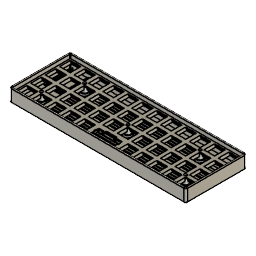
Like Planck (Autodesk Fusion 360 design; units mm, degrees)
Autodesk Fusion 360 part; units mm, degrees
note: some values were not read from the file. Set by a fixed rule: which sketch regions a step uses.
(part 1 of 2)
sketch "Base Sketch" plane through (0, 0, 0) normal (0, 0, 1) x (1, 0, 0)
  line L0 (99.1182, 9.2838) -> (99.1182, 3.0138)
  line L1 (104.144, 3.0138) -> (105.869, 3.0138)
  line L2 (105.869, 15.3128) -> (99.1182, 15.3128)
  line L3 (107.395, 2.7836) -> (121.394, 2.7836)
  line L4 (129.669, 12.0826) -> (129.669, 15.3128)
  line L5 (98.2941, 9.2838) -> (99.1182, 9.2838)
  line L6 (107.395, 16.7831) -> (107.395, 12.0826)
  line L7 (129.669, 9.2838) -> (130.495, 9.2838)
  line L8 (99.1182, 3.0138) -> (100.845, 3.0138)
  line L9 (130.495, 9.2838) -> (130.495, 12.0826)
  line L10 (0.0951, 0.2577) -> (0.0951, 76.4575)
  line L11 (122.92, 12.0826) -> (121.394, 12.0826)
  line L12 (2.6197, 16.7831) -> (16.6192, 16.7831)
  line L13 (121.394, 16.7831) -> (107.395, 16.7831)
  line L14 (105.869, 7.4827) -> (107.395, 7.4827)
  line L15 (228.695, 76.4575) -> (228.695, 0.2577)
  line L16 (105.869, 12.0826) -> (105.869, 15.3128)
  line L17 (98.2941, 12.0826) -> (98.2941, 9.2838)
  line L18 (107.395, 12.0826) -> (105.869, 12.0826)
  line L19 (121.394, 2.7836) -> (121.394, 7.4827)
  line L20 (124.645, 3.0138) -> (124.645, 1.8135)
  line L21 (99.1182, 12.0826) -> (98.2941, 12.0826)
  line L22 (127.944, 1.8135) -> (127.944, 3.0138)
  line L23 (121.394, 7.4827) -> (122.92, 7.4827)
  line L24 (122.92, 3.0138) -> (124.645, 3.0138)
  line L25 (100.845, 1.8135) -> (104.144, 1.8135)
  line L26 (124.645, 1.8135) -> (127.944, 1.8135)
  line L27 (155.02, 16.7831) -> (169.019, 16.7831)
  line L28 (149.969, 2.7836) -> (135.97, 2.7836)
  line L29 (35.669, 2.7836) -> (21.6697, 2.7836)
  line L30 (226.169, 2.7836) -> (212.17, 2.7836)
  line L31 (127.944, 3.0138) -> (129.669, 3.0138)
  line L32 (21.6697, 35.833) -> (35.669, 35.833)
  line L33 (40.7197, 35.833) -> (54.719, 35.833)
  line L34 (16.6192, 21.8336) -> (2.6196, 21.8336)
  line L35 (2.6197, 2.7836) -> (2.6197, 16.7831)
  line L36 (104.144, 1.8135) -> (104.144, 3.0138)
  line L37 (130.495, 12.0826) -> (129.669, 12.0826)
  line L38 (35.669, 16.7831) -> (35.669, 2.7836)
  line L39 (59.7697, 16.7831) -> (73.769, 16.7831)
  line L40 (0.0951, 76.4575) -> (228.695, 76.4575)
  line L41 (121.394, 12.0826) -> (121.394, 16.7831)
  line L42 (188.069, 2.7836) -> (174.07, 2.7836)
  line L43 (228.695, 0.2577) -> (0.0951, 0.2577)
  line L44 (135.97, 16.7831) -> (149.969, 16.7831)
  line L45 (59.7697, 2.7836) -> (59.7697, 16.7831)
  line L46 (169.019, 2.7836) -> (155.02, 2.7836)
  line L47 (116.918, 35.833) -> (130.919, 35.833)
  line L48 (149.969, 21.8336) -> (135.97, 21.8336)
  line L49 (107.395, 7.4827) -> (107.395, 2.7836)
  line L50 (54.719, 35.833) -> (54.719, 21.8336)
  line L51 (78.8197, 16.7831) -> (92.819, 16.7831)
  line L52 (207.119, 16.7831) -> (207.119, 2.7836)
  line L53 (73.769, 21.8336) -> (59.7697, 21.8336)
  line L54 (135.97, 21.8336) -> (135.97, 35.833)
  line L55 (207.119, 21.8336) -> (193.12, 21.8336)
  line L56 (122.92, 15.3128) -> (122.92, 12.0826)
  line L57 (16.6192, 2.7836) -> (2.6196, 2.7836)
  line L58 (193.12, 16.7831) -> (207.119, 16.7831)
  line L59 (188.069, 16.7831) -> (188.069, 2.7836)
  line L60 (212.17, 2.7836) -> (212.17, 16.7831)
  line L61 (130.919, 35.833) -> (130.919, 21.8336)
  line L62 (212.17, 16.7831) -> (226.169, 16.7831)
  line L63 (129.669, 3.0138) -> (129.669, 9.2838)
  line L64 (54.719, 21.8336) -> (40.7197, 21.8336)
  line L65 (16.6192, 16.7831) -> (16.6192, 2.7836)
  line L66 (40.7197, 2.7836) -> (40.7197, 16.7831)
  line L67 (100.845, 3.0138) -> (100.845, 1.8135)
  line L68 (135.97, 2.7836) -> (135.97, 16.7831)
  line L69 (92.819, 2.7836) -> (78.8197, 2.7836)
  line L70 (174.07, 16.7831) -> (188.069, 16.7831)
  line L71 (35.669, 35.833) -> (35.669, 21.8336)
  line L72 (92.819, 16.7831) -> (92.819, 2.7836)
  line L73 (155.02, 2.7836) -> (155.02, 16.7831)
  line L74 (129.669, 15.3128) -> (122.92, 15.3128)
  line L75 (73.769, 35.833) -> (73.769, 21.8336)
  line L76 (169.019, 16.7831) -> (169.019, 2.7836)
  line L77 (54.719, 2.7836) -> (40.7197, 2.7836)
  line L78 (59.7697, 35.833) -> (73.769, 35.833)
  line L79 (99.1182, 15.3128) -> (99.1182, 12.0826)
  line L80 (73.769, 2.7836) -> (59.7697, 2.7836)
  line L81 (122.92, 7.4827) -> (122.92, 3.0138)
  line L82 (105.869, 3.0138) -> (105.869, 7.4827)
  line L83 (21.6697, 16.7831) -> (35.669, 16.7831)
  line L84 (54.719, 16.7831) -> (54.719, 2.7836)
  line L85 (78.8197, 2.7836) -> (78.8197, 16.7831)
  line L86 (21.6697, 2.7836) -> (21.6697, 16.7831)
  line L87 (149.969, 16.7831) -> (149.969, 2.7836)
  line L88 (40.7197, 16.7831) -> (54.719, 16.7831)
  line L89 (73.769, 16.7831) -> (73.769, 2.7836)
  line L90 (174.07, 2.7836) -> (174.07, 16.7831)
  line L91 (21.6697, 40.8838) -> (21.6697, 54.8831)
  line L92 (40.7197, 21.8336) -> (40.7197, 35.833)
  line L93 (97.8683, 35.833) -> (111.869, 35.833)
  line L94 (116.918, 21.8336) -> (116.918, 35.833)
  line L95 (130.919, 54.8831) -> (130.919, 40.8838)
  line L96 (21.6697, 73.9331) -> (35.669, 73.9331)
  line L97 (155.02, 35.833) -> (169.019, 35.833)
  line L98 (116.918, 40.8838) -> (116.918, 54.8831)
  line L99 (78.8197, 59.9338) -> (78.8197, 73.9331)
  line L100 (111.869, 73.9331) -> (111.869, 59.9338)
  line L101 (155.02, 54.8831) -> (169.019, 54.8831)
  line L102 (174.07, 35.833) -> (188.069, 35.833)
  line L103 (78.8197, 21.8336) -> (78.8197, 35.833)
  line L104 (193.12, 21.8336) -> (193.12, 35.833)
  line L105 (59.7697, 21.8336) -> (59.7697, 35.833)
  line L106 (2.6197, 21.8336) -> (2.6197, 35.833)
  line L107 (35.669, 21.8336) -> (21.6697, 21.8336)
  line L108 (149.969, 35.833) -> (149.969, 21.8336)
  line L109 (2.6197, 54.8831) -> (16.6192, 54.8831)
  line L110 (169.019, 54.8831) -> (169.019, 40.8838)
  line L111 (78.8197, 73.9331) -> (92.819, 73.9331)
  line L112 (92.819, 59.9338) -> (78.8197, 59.9338)
  line L113 (169.019, 21.8336) -> (155.02, 21.8336)
  line L114 (226.169, 35.833) -> (226.169, 21.8336)
  line L115 (188.069, 21.8336) -> (174.07, 21.8336)
  line L116 (35.669, 40.8838) -> (21.6697, 40.8838)
  line L117 (35.669, 54.8831) -> (35.669, 40.8838)
  line L118 (188.069, 35.833) -> (188.069, 21.8336)
  line L119 (21.6697, 54.8831) -> (35.669, 54.8831)
  line L120 (111.869, 21.8336) -> (97.8683, 21.8336)
  line L121 (169.019, 35.833) -> (169.019, 21.8336)
  line L122 (130.919, 21.8336) -> (116.918, 21.8336)
  line L123 (193.12, 2.7836) -> (193.12, 16.7831)
  line L124 (92.819, 21.8336) -> (78.8197, 21.8336)
  line L125 (92.819, 35.833) -> (92.819, 21.8336)
  line L126 (73.769, 59.9338) -> (59.7697, 59.9338)
  line L127 (59.7697, 54.8831) -> (73.769, 54.8831)
  line L128 (207.119, 35.833) -> (207.119, 21.8336)
  line L129 (73.769, 40.8838) -> (59.7697, 40.8838)
  line L130 (92.819, 73.9331) -> (92.819, 59.9338)
  line L131 (40.7197, 73.9331) -> (54.719, 73.9331)
  line L132 (54.719, 54.8831) -> (54.719, 40.8838)
  line L133 (226.169, 21.8336) -> (212.17, 21.8336)
  line L134 (16.6192, 54.8831) -> (16.6192, 40.8838)
  line L135 (111.869, 35.833) -> (111.869, 21.8336)
  line L136 (16.6192, 40.8838) -> (2.6196, 40.8838)
  line L137 (193.12, 35.833) -> (207.119, 35.833)
  line L138 (226.169, 16.7831) -> (226.169, 2.7836)
  line L139 (212.17, 35.833) -> (226.169, 35.833)
  line L140 (2.6197, 35.833) -> (16.6192, 35.833)
  line L141 (207.119, 2.7836) -> (193.12, 2.7836)
  line L142 (149.969, 40.8838) -> (135.97, 40.8838)
  line L143 (16.6192, 35.833) -> (16.6192, 21.8336)
  line L144 (212.17, 21.8336) -> (212.17, 35.833)
  line L145 (21.6697, 21.8336) -> (21.6697, 35.833)
  line L146 (155.02, 21.8336) -> (155.02, 35.833)
  line L147 (174.07, 21.8336) -> (174.07, 35.833)
  line L148 (97.8683, 21.8336) -> (97.8683, 35.833)
  line L149 (78.8197, 35.833) -> (92.819, 35.833)
  line L150 (40.7197, 54.8831) -> (54.719, 54.8831)
  line L151 (97.8683, 73.9331) -> (111.869, 73.9331)
  line L152 (2.6197, 40.8838) -> (2.6197, 54.8831)
  line L153 (92.819, 54.8831) -> (92.819, 40.8838)
  line L154 (135.97, 35.833) -> (149.969, 35.833)
  line L155 (73.769, 54.8831) -> (73.769, 40.8838)
  line L156 (135.97, 54.8831) -> (149.969, 54.8831)
  line L157 (59.7697, 73.9331) -> (73.769, 73.9331)
  line L158 (40.7197, 40.8838) -> (40.7197, 54.8831)
  line L159 (21.6697, 59.9338) -> (21.6697, 73.9331)
  line L160 (212.17, 73.9331) -> (226.169, 73.9331)
  line L161 (111.869, 54.8831) -> (111.869, 40.8838)
  line L162 (193.12, 59.9338) -> (193.12, 73.9331)
  line L163 (212.17, 40.8838) -> (212.17, 54.8831)
  line L164 (2.6197, 73.9331) -> (16.6192, 73.9331)
  line L165 (97.8683, 59.9338) -> (97.8683, 73.9331)
  line L166 (59.7697, 40.8838) -> (59.7697, 54.8831)
  line L167 (111.869, 59.9338) -> (97.8683, 59.9338)
  line L168 (174.07, 40.8838) -> (174.07, 54.8831)
  line L169 (97.8683, 40.8838) -> (97.8683, 54.8831)
  line L170 (16.6192, 59.9338) -> (2.6196, 59.9338)
  line L171 (135.97, 40.8838) -> (135.97, 54.8831)
  line L172 (193.12, 40.8838) -> (193.12, 54.8831)
  line L173 (2.6197, 59.9338) -> (2.6197, 73.9331)
  line L174 (40.7197, 59.9338) -> (40.7197, 73.9331)
  line L175 (130.919, 73.9331) -> (130.919, 59.9338)
  line L176 (174.07, 59.9338) -> (174.07, 73.9331)
  line L177 (35.669, 59.9338) -> (21.6697, 59.9338)
  line L178 (149.969, 59.9338) -> (135.97, 59.9338)
  line L179 (78.8197, 54.8831) -> (92.819, 54.8831)
  line L180 (155.02, 40.8838) -> (155.02, 54.8831)
  line L181 (54.719, 59.9338) -> (40.7197, 59.9338)
  line L182 (149.969, 73.9331) -> (149.969, 59.9338)
  line L183 (207.119, 59.9338) -> (193.12, 59.9338)
  line L184 (207.119, 40.8838) -> (193.12, 40.8838)
  line L185 (188.069, 54.8831) -> (188.069, 40.8838)
  line L186 (226.169, 40.8838) -> (212.17, 40.8838)
  line L187 (188.069, 73.9331) -> (188.069, 59.9338)
  line L188 (111.869, 40.8838) -> (97.8683, 40.8838)
  line L189 (116.918, 59.9338) -> (116.918, 73.9331)
  line L190 (130.919, 40.8838) -> (116.918, 40.8838)
  line L191 (116.918, 54.8831) -> (130.919, 54.8831)
  line L192 (174.07, 54.8831) -> (188.069, 54.8831)
  line L193 (212.17, 54.8831) -> (226.169, 54.8831)
  line L194 (149.969, 54.8831) -> (149.969, 40.8838)
  line L195 (92.819, 40.8838) -> (78.8197, 40.8838)
  line L196 (130.919, 59.9338) -> (116.918, 59.9338)
  line L197 (155.02, 59.9338) -> (155.02, 73.9331)
  line L198 (188.069, 40.8838) -> (174.07, 40.8838)
  line L199 (135.97, 59.9338) -> (135.97, 73.9331)
  line L200 (135.97, 73.9331) -> (149.969, 73.9331)
  line L201 (116.918, 73.9331) -> (130.919, 73.9331)
  line L202 (73.769, 73.9331) -> (73.769, 59.9338)
  line L203 (226.169, 54.8831) -> (226.169, 40.8838)
  line L204 (193.12, 54.8831) -> (207.119, 54.8831)
  line L205 (54.719, 40.8838) -> (40.7197, 40.8838)
  line L206 (226.169, 73.9331) -> (226.169, 59.9338)
  line L207 (35.669, 73.9331) -> (35.669, 59.9338)
  line L208 (188.069, 59.9338) -> (174.07, 59.9338)
  line L209 (78.8197, 40.8838) -> (78.8197, 54.8831)
  line L210 (16.6192, 73.9331) -> (16.6192, 59.9338)
  line L211 (174.07, 73.9331) -> (188.069, 73.9331)
  line L212 (207.119, 54.8831) -> (207.119, 40.8838)
  line L213 (97.8683, 54.8831) -> (111.869, 54.8831)
  line L214 (59.7697, 59.9338) -> (59.7697, 73.9331)
  line L215 (169.019, 59.9338) -> (155.02, 59.9338)
  line L216 (169.019, 40.8838) -> (155.02, 40.8838)
  line L217 (193.12, 73.9331) -> (207.119, 73.9331)
  line L218 (54.719, 73.9331) -> (54.719, 59.9338)
  line L219 (169.019, 73.9331) -> (169.019, 59.9338)
  line L220 (212.17, 59.9338) -> (212.17, 73.9331)
  line L221 (207.119, 73.9331) -> (207.119, 59.9338)
  line L222 (155.02, 73.9331) -> (169.019, 73.9331)
  line L223 (226.169, 59.9338) -> (212.17, 59.9338)
  line L224 (-0.2049, 76.7575) -> (228.995, 76.7575)
  line L225 (228.995, 76.7575) -> (228.995, -0.0423)
  line L226 (228.995, -0.0423) -> (-0.2049, -0.0423)
  line L227 (-0.2049, -0.0423) -> (-0.2049, 76.7575)
  line L228 (-2.0049, 78.5575) -> (230.795, 78.5575)
  line L229 (230.795, 78.5575) -> (230.795, -1.8423)
  line L230 (230.795, -1.8423) -> (-2.0049, -1.8423)
  line L231 (-2.0049, -1.8423) -> (-2.0049, 78.5575)
  line L232 (212.17, 16.7831) -> (207.119, 21.8336) construction
  line L233 (207.119, 16.7831) -> (212.17, 21.8336) construction
  line L234 (111.869, 35.833) -> (116.918, 40.8838) construction
  line L235 (116.918, 35.833) -> (111.869, 40.8838) construction
  line L236 (16.6192, 16.7831) -> (21.6697, 21.8336) construction
  line L237 (21.6697, 16.7831) -> (16.6192, 21.8336) construction
  circle A0 centre (209.6445, 19.3084) radius 3.5714
  circle A1 centre (114.3935, 38.3584) radius 3.5708
  circle A2 centre (19.1445, 19.3084) radius 3.5712
  line L238 (35.669, 59.9338) -> (40.7197, 54.8831) construction
  line L239 (40.7197, 59.9338) -> (35.669, 54.8831) construction
  line L240 (193.12, 59.9338) -> (188.069, 54.8831) construction
  line L241 (188.069, 59.9338) -> (193.12, 54.8831) construction
  circle A3 centre (190.5945, 57.4085) radius 3.5715
  circle A4 centre (38.1944, 57.4085) radius 3.5714
  circle A5 centre (38.1944, 57.4085) radius 1
  circle A6 centre (19.1445, 19.3084) radius 1
  circle A7 centre (114.3935, 38.3584) radius 1
  circle A8 centre (190.5945, 57.4085) radius 1
  circle A9 centre (209.6445, 19.3084) radius 1
  line L242 (2.6197, 73.9331) -> (2.6197, 0.2577)
  line L243 (2.6197, 73.9331) -> (2.6197, 76.4575)
  line L244 (16.6192, 73.9331) -> (16.6192, 0.2577)
  line L245 (35.669, 73.9331) -> (35.669, 0.2577)
  line L246 (54.719, 73.9331) -> (54.719, 0.2577)
  line L247 (73.769, 73.9331) -> (73.769, 0.2577)
  line L248 (92.819, 73.9331) -> (92.819, 0.2577)
  line L249 (111.869, 73.9331) -> (111.869, 16.7831)
  line L250 (130.919, 73.9331) -> (130.919, 0.2577)
  line L251 (149.969, 73.9331) -> (149.969, 0.2577)
  line L252 (169.019, 73.9331) -> (169.019, 0.2577)
  line L253 (188.069, 73.9331) -> (188.069, 0.2577)
  line L254 (207.119, 73.9331) -> (207.119, 0.2577)
  line L255 (226.169, 73.9331) -> (226.169, 0.2577)
  line L256 (212.17, 73.9331) -> (212.17, 0.2577)
  line L257 (193.12, 73.9331) -> (193.12, 0.2577)
  line L258 (174.07, 73.9331) -> (174.07, 0.2577)
  line L259 (155.02, 73.9331) -> (155.02, 0.2577)
  line L260 (135.97, 73.9331) -> (135.97, 0.2577)
  line L261 (116.918, 73.9331) -> (116.918, 16.7831)
  line L262 (97.8683, 73.9331) -> (97.8683, 0.2577)
  line L263 (78.8197, 73.9331) -> (78.8197, 0.2577)
  line L264 (59.7697, 73.9331) -> (59.7697, 0.2577)
  line L265 (40.7197, 73.9331) -> (40.7197, 0.2577)
  line L266 (21.6697, 73.9331) -> (21.6697, 0.2577)
  line L267 (16.6192, 73.9331) -> (16.6192, 76.4575)
  line L268 (21.6697, 76.4575) -> (21.6697, 73.9331)
  line L269 (35.669, 76.4575) -> (35.669, 73.9331)
  line L270 (40.7197, 76.4575) -> (40.7197, 73.9331)
  line L271 (54.719, 76.4575) -> (54.719, 73.9331)
  line L272 (59.7697, 76.4575) -> (59.7697, 73.9331)
  line L273 (73.769, 76.4575) -> (73.769, 73.9331)
  line L274 (78.8197, 76.4575) -> (78.8197, 73.9331)
  line L275 (92.819, 76.4575) -> (92.819, 73.9331)
  line L276 (97.8683, 76.4575) -> (97.8683, 73.9331)
  line L277 (111.869, 76.4575) -> (111.869, 73.9331)
  line L278 (116.918, 76.4575) -> (116.918, 73.9331)
  line L279 (130.919, 76.4575) -> (130.919, 73.9331)
  line L280 (135.97, 76.4575) -> (135.97, 73.9331)
  line L281 (149.969, 76.4575) -> (149.969, 73.9331)
  line L282 (155.02, 76.4575) -> (155.02, 73.9331)
  line L283 (169.019, 76.4575) -> (169.019, 73.9331)
  line L284 (174.07, 76.4575) -> (174.07, 73.9331)
  line L285 (188.069, 76.4575) -> (188.069, 73.9331)
  line L286 (193.12, 76.4575) -> (193.12, 73.9331)
  line L287 (207.119, 76.4575) -> (207.119, 73.9331)
  line L288 (212.17, 76.4575) -> (212.17, 73.9331)
  line L289 (226.169, 76.4575) -> (226.169, 73.9331)
  line L290 (2.6197, 75.1331) -> (226.169, 75.1331)
  line L291 (226.169, 58.7338) -> (2.6197, 58.7338)
  line L292 (2.6197, 56.0831) -> (226.169, 56.0831)
  line L293 (226.169, 39.6838) -> (2.6197, 39.6838)
  line L294 (2.6197, 37.033) -> (226.169, 37.033)
  line L295 (226.169, 20.6336) -> (2.6197, 20.6336)
  line L296 (2.6197, 17.9831) -> (226.169, 17.9831)
  line L297 (226.169, 1.5836) -> (2.6197, 1.5836)
  line L298 (107.395, 16.7831) -> (107.395, 21.8336)
  line L299 (121.394, 16.7831) -> (121.394, 21.8336)
  line L300 (121.394, 2.7836) -> (121.394, 0.2577)
  line L301 (107.395, 2.7836) -> (107.395, 0.2577)
  circle A10 centre (38.1944, 57.4085) radius 4.25
  circle A11 centre (19.1445, 19.3084) radius 4.25
  circle A12 centre (114.3935, 38.3584) radius 4.25
  circle A13 centre (190.5945, 57.4085) radius 4.25
  circle A14 centre (209.6445, 19.3084) radius 4.25
  dimension "d7" = 1.8
  dimension "d8" = 1.8
  dimension "d9" = 1.8
  dimension "d10" = 1.8
  dimension "d62" = 2
  dimension "d63" = 2
  dimension "d64" = 2
  dimension "d65" = 2
  dimension "d66" = 2
  dimension "d83" = 1.2
  dimension "d84" = 1.2
  dimension "d85" = 1.2
  dimension "d87" = 1.2
  dimension "d88" = 1.2
  dimension "d89" = 1.2
  dimension "d90" = 1.2
  dimension "d91" = 1.2
  dimension "d94" = 8.5
  dimension "d95" = 8.5
  dimension "d96" = 8.5
  dimension "d97" = 8.5
  dimension "d98" = 8.5
  constraint horizontal L224
  constraint vertical L225
  constraint horizontal L226
  constraint vertical L227
  constraint horizontal L228
  constraint vertical L229
  constraint horizontal L230
  constraint vertical L231
  constraint midpoint L233 A0.centre
  constraint coincident L55.start A0
  constraint midpoint L235 A1.centre
  constraint coincident L161.end A1
  constraint midpoint L236 A2.centre
  constraint coincident L34.start A2
  constraint midpoint L241 A3.centre
  constraint coincident L172.end A3
  constraint midpoint L239 A4.centre
  constraint coincident L150.start A4
  constraint concentric A4 A5
  constraint concentric A2 A6
  constraint concentric A1 A7
  constraint concentric A3 A8
  constraint concentric A0 A9
  constraint coincident L43 L242.end
  constraint perpendicular L43 L242
  constraint coincident L40 L243.end
  constraint coincident L43 L244.end
  constraint coincident L43 L245.end
  constraint coincident L43 L246.end
  constraint coincident L43 L247.end
  constraint coincident L13 L249.end
  constraint perpendicular L13 L249
  constraint coincident L43 L250.end
  constraint coincident L43 L251.end
  constraint coincident L43 L252.end
  constraint coincident L43 L253.end
  constraint coincident L43 L254.end
  constraint coincident L43 L255.end
  constraint coincident L43 L256.end
  constraint coincident L43 L257.end
  constraint perpendicular L42 L258
  constraint coincident L43 L259.end
  constraint coincident L43 L260.end
  constraint coincident L13 L261.end
  constraint coincident L43 L262.end
  constraint coincident L43 L263.end
  constraint coincident L40 L267.end
  constraint perpendicular L40 L267
  constraint coincident L40 L268.start
  constraint coincident L40 L269.start
  constraint coincident L40 L270.start
  constraint coincident L40 L271.start
  constraint coincident L40 L272.start
  constraint coincident L40 L273.start
  constraint coincident L40 L274.start
  constraint coincident L40 L275.start
  constraint coincident L40 L276.start
  constraint coincident L40 L277.start
  constraint coincident L40 L278.start
  constraint coincident L40 L279.start
  constraint coincident L40 L280.start
  constraint coincident L40 L281.start
  constraint coincident L40 L282.start
  constraint coincident L40 L283.start
  constraint coincident L40 L284.start
  constraint coincident L40 L285.start
  constraint coincident L40 L286.start
  constraint coincident L40 L287.start
  constraint coincident L40 L288.start
  constraint coincident L40 L289.start
  constraint coincident L243 L290.start
  constraint coincident L289 L290.end
  constraint perpendicular L289 L290
  constraint coincident L255 L291.start
  constraint coincident L242 L291.end
  constraint perpendicular L242 L291
  constraint coincident L242 L292.start
  constraint coincident L255 L292.end
  constraint perpendicular L255 L292
  constraint coincident L255 L293.start
  constraint perpendicular L242 L293
  constraint coincident L255 L295.start
  constraint coincident L242 L295.end
  constraint perpendicular L242 L295
  constraint coincident L242 L296.start
  constraint coincident L255 L296.end
  constraint perpendicular L255 L296
  constraint coincident L255 L297.start
  constraint perpendicular L242 L297
  constraint coincident L120 L298.end
  constraint coincident L122 L299.end
  constraint coincident L43 L300.end
  constraint perpendicular L43 L300
  constraint coincident L43 L301.end
  constraint perpendicular L43 L301
  constraint concentric A4 A10
  constraint concentric A2 A11
  constraint concentric A1 A12
  constraint concentric A8 A13
  constraint concentric A0 A14
  measures "d7" distance of L227 L231
  measures "d8" distance of L224 L228
  measures "d9" distance of L225 L229
  measures "d10" distance of L226 L230
  measures "d62" diameter of A5
  measures "d63" diameter of A6
  measures "d64" diameter of A7
  measures "d65" diameter of A8
  measures "d66" diameter of A9
  measures "d83" distance of L69 L297
  measures "d84" distance of L51 L296
  measures "d85" distance of L124 L295
  measures "d87" distance of L149 L294
  measures "d88" distance of L195 L293
  measures "d89" distance of L179 L292
  measures "d90" distance of L112 L291
  measures "d91" distance of L111 L290
  measures "d94" diameter of A10
  measures "d95" diameter of A11
  measures "d96" diameter of A12
  measures "d97" diameter of A13
  measures "d98" diameter of A14
extrude "Extrude1" add sketch "Base Sketch" along normal blind 1.6 contours L0 L1 L2 L5 L6 L8 L14 L16 L17 L18 L21 L25 L36 L49 L67 L79 L82 L262 L296 L297 L298 L301 | L13 L249 L296 L298 | L3 L297 L300 L301 | L13 L249 L261 L296 | L249 L295 L296 L298 | L262 L295 L296 L298 | L4 L7 L9 L11 L19 L20 L22 L23 L24 L26 L31 L37 L41 L56 L63 L74 L81 L250 L296 L297 L299 L300 | L43 L262 L297 L301 | L43 L297 L300 L301 | L13 L261 L296 L299 | L249 L261 L295 L296 | L248 L262 L295 L296 | L72 L248 L262 L296 L297 | L120 L249 L295 L298 | L120 L262 L295 L298 | L43 L250 L297 L300 | L43 L248 L262 L297 | L261 L295 L296 L299 | L94 L135 L249 L261 L295 A12 | L125 L148 L248 L262 L294 L295 | L248 L263 L295 L296 | L51 L248 L263 L296 | L43 L250 L260 L297 | L68 L250 L260 L296 L297 | L69 L248 L263 L297 | L43 L248 L263 L297 | L250 L295 L296 L299 | L122 L261 L295 L299 | L124 L248 L263 L295 | L247 L263 L295 L296 | L85 L89 L247 L263 L296 L297 | L250 L260 L295 L296 | L43 L251 L260 L297 | L28 L251 L260 L297 | L43 L247 L263 L297 | L122 L250 L295 L299 | L94 L135 A1 L249 L261 A12 | L93 L262 L294 A12 | L75 L103 L247 L263 L294 L295 | L247 L264 L295 L296 | L39 L247 L264 L296 | L54 L61 L250 L260 L294 L295 | L44 L251 L260 L296 | L251 L260 L295 L296 | L43 L251 L259 L297 | L73 L87 L251 L259 L296 L297 | L80 L247 L264 L297 | L43 L247 L264 L297 | A1 L249 L261 L294 | L93 A1 L294 A12 | A1 L249 L294 | L248 L262 L293 L294 | L262 L293 L294 A12 | L149 L248 L263 L294 | L53 L247 L264 L295 | L246 L264 L295 L296 | L45 L84 L246 L264 L296 L297 | L48 L251 L260 L295 | L251 L259 L295 L296 | L43 L252 L259 L297 | L46 L252 L259 L297 | L43 L246 L264 L297 | L47 A1 L294 A12 | A1 L261 L294 | L47 L250 L294 A12 | A1 L293 L294 A12 | A1 L249 L293 L294 | L249 L261 L293 L294 | L153 L169 L248 L262 L292 L293 | L188 L262 L293 A12 | L248 L263 L293 L294 | L50 L105 L246 L264 L294 L295 | L246 L265 L295 L296 | L88 L246 L265 L296 | L108 L146 L251 L259 L294 L295 | L27 L252 L259 L296 | L252 L259 L295 L296 | L43 L252 L258 L297 | L76 L90 L252 L258 L296 L297 | L77 L246 L265 L297 | L43 L246 L265 L297 | A1 L261 L293 L294 | A1 L293 L294 A12 | L250 L293 L294 A12 | L188 A1 L293 A12 | A1 L249 L293 | A1 L249 L261 L293 | L195 L248 L263 L293 | L247 L263 L293 L294 | L78 L247 L264 L294 | L64 L246 L265 L295 | L245 L265 L295 L296 | L38 L66 L245 L265 L296 L297 | L250 L260 L293 L294 | L154 L251 L260 L294 | L113 L252 L259 L295 | L252 L258 L295 L296 | L43 L253 L258 L297 | L42 L253 L258 L297 | L43 L245 L265 L297 | A1 L261 L293 | L98 L161 A1 L249 L261 A12 | L213 L249 L262 L292 | L155 L209 L247 L263 L292 L293 | L247 L264 L293 L294 | L71 L92 L245 L265 L294 L295 | L245 L295 L296 A11 | L83 L245 L296 A11 | L190 L250 L293 A12 | L95 L171 L250 L260 L292 L293 | L251 L260 L293 L294 | L121 L147 L252 L258 L294 L295 | L70 L253 L258 L296 | L253 L258 L295 L296 | L43 L253 L257 L297 | L59 L123 L253 L257 L296 L297 | L29 L245 L266 L297 | L43 L245 L266 L297 | L190 A1 L293 A12 | L98 L161 L249 L261 L292 A12 | L248 L262 L291 L292 | L249 L262 L291 L292 | L179 L248 L263 L292 | L129 L247 L264 L293 | L246 L264 L293 L294 | L33 L246 L265 L294 | L107 L245 L295 A11 | L83 A2 L296 A11 | A2 L295 L296 A11 | L142 L251 L260 L293 | L251 L259 L293 L294 | L97 L252 L259 L294 | L115 L253 L258 L295 | L253 L257 L295 L296 | L43 L254 L257 L297 | L141 L254 L257 L297 | L65 L86 L244 L266 L297 A11 | L43 L244 L266 L297 | L249 L261 L291 L292 | L130 L165 L248 L262 L275 L276 L290 L291 | L167 L249 L262 L291 | L248 L263 L291 L292 | L132 L166 L246 L264 L292 L293 | L246 L265 L293 L294 | L107 A2 L295 A11 | A2 L266 L295 L296 | A2 L266 L296 | L191 L250 L261 L292 | L180 L194 L251 L259 L292 L293 | L252 L259 L293 L294 | L104 L118 L253 L257 L294 L295 | L58 L257 L296 A14 | L257 L295 L296 A14 | L43 L254 L256 L297 | L52 L60 L254 L256 L297 A14 | L57 L242 L244 L297 | L43 L242 L244 L297 | L100 L189 L249 L261 L277 L278 L290 L291 | L250 L261 L291 L292 | L112 L248 L263 L291 | L247 L263 L291 L292 | L127 L247 L264 L292 | L205 L246 L265 L293 | L245 L265 L293 L294 | L32 L245 L266 L294 | A2 L266 L295 | L65 L86 A2 L244 L266 A11 | A2 L244 L266 L296 | L244 L266 L295 L296 | L250 L260 L291 L292 | L156 L251 L260 L292 | L216 L252 L259 L293 | L252 L258 L293 L294 | L102 L253 L258 L294 | L55 L257 L295 A14 | A0 L295 L296 A14 | L58 A0 L296 A14 | L43 L255 L256 L297 | L30 L255 L256 L297 | L10 L35 L40 L43 L106 L152 L173 L242 L243 | L196 L250 L261 L291 | L151 L276 L277 L290 | L99 L202 L247 L263 L273 L274 L290 L291 | L247 L264 L291 L292 | L117 L158 L245 L265 L293 A10 | L245 L266 L293 L294 | L143 L145 L244 L266 L294 A11 | L143 L145 A2 L244 L266 A11 | A2 L244 L266 L295 | L12 A2 L296 A11 | A2 L244 L296 | A2 L244 L295 L296 | L175 L199 L250 L260 L279 L280 L290 L291 | L251 L260 L291 L292 | L110 L168 L252 L258 L292 L293 | L253 L258 L293 L294 | L55 A0 L295 A14 | A0 L254 L296 | A0 L254 L295 L296 | L52 L60 A0 L254 L256 A14 | L15 L40 L43 L114 L138 L203 L206 L255 L289 | L40 L275 L276 L290 | L40 L276 L277 L290 | L111 L274 L275 L290 | L126 L247 L264 L291 | L246 L264 L291 L292 | L150 L246 L292 A10 | L116 L245 L266 L293 | L244 L266 L293 L294 | L34 A2 L295 A11 | A2 L244 L295 | L12 L242 L296 A11 | A2 L295 L296 A11 | L178 L251 L260 L291 | L251 L259 L291 L292 | L101 L252 L259 L292 | L198 L253 L258 L293 | L253 L257 L293 L294 | L137 L254 L257 L294 | A0 L254 L295 | A0 L254 L256 L296 | L254 L256 L295 L296 | L40 L277 L278 L290 | L201 L278 L279 L290 | L40 L274 L275 L290 | L214 L218 L246 L264 L271 L272 L290 L291 | L246 L291 L292 A10 | L150 A4 L292 A10 | L117 L158 A4 L245 L265 A10 | L91 L134 L244 L266 L292 L293 | L242 L244 L293 L294 | L140 L242 L244 L294 | L34 L242 L295 A11 | L242 L295 L296 A11 | L182 L197 L251 L259 L281 L282 L290 L291 | L252 L259 L291 L292 | L172 L185 L253 L257 L293 A13 | L254 L257 L293 L294 | L128 L144 A0 L254 L256 A14 | A0 L254 L256 L295 | L128 L144 L254 L256 L294 A14 | L62 A0 L296 A14 | A0 L256 L296 | A0 L256 L295 L296 | L62 L255 L296 A14 | L40 L278 L279 L290 | L40 L273 L274 L290 | L157 L272 L273 L290 | L181 L246 L291 A10 | A4 L291 L292 A10 | A4 L265 L292 | A4 L245 L265 L292 | L136 L242 L244 L293 | L40 L279 L280 L290 | L200 L280 L281 L290 | L215 L252 L259 L291 | L252 L258 L291 L292 | L192 L258 L292 A13 | L184 L254 L257 L293 | L254 L256 L293 L294 | L133 A0 L295 A14 | A0 L256 L295 | A0 L295 L296 A14 | L255 L295 L296 A14 | L40 L243 L267 L290 | L40 L272 L273 L290 | L181 A4 L291 A10 | A4 L265 L291 L292 | L119 A4 L292 A10 | A4 L245 L292 | L245 L265 L291 L292 | L119 L266 L292 A10 | L40 L280 L281 L290 | L176 L219 L252 L258 L283 L284 L290 L291 | L258 L291 L292 A13 | L192 A3 L292 A13 | L172 L185 A3 L253 L257 A13 | L163 L212 L254 L256 L292 L293 | L139 L255 L256 L294 | L255 L256 L293 L294 | L133 L255 L295 A14 | L40 L288 L289 L290 | L40 L267 L268 L290 | L164 L243 L267 L290 | L40 L271 L272 L290 | L131 L270 L271 L290 | A4 L265 L291 | A4 L291 L292 A10 | A4 L245 L291 L292 | A4 L245 L265 L291 | L266 L291 L292 A10 | L244 L266 L291 L292 | L109 L242 L244 L292 | L40 L281 L282 L290 | L222 L282 L283 L290 | L208 L258 L291 A13 | A3 L291 L292 A13 | A3 L253 L257 L292 | A3 L253 L292 | L186 L255 L256 L293 | L40 L287 L288 L290 | L160 L288 L289 L290 | L40 L268 L269 L290 | L159 L210 L244 L266 L267 L268 L290 L291 | L40 L270 L271 L290 | L174 L207 A4 L245 L265 A10 | L174 L207 L245 L265 L269 L270 L290 A10 | L177 A4 L291 A10 | A4 L245 L291 | L177 L266 L291 A10 | L242 L244 L291 L292 | L40 L282 L283 L290 | L208 A3 L291 A13 | A3 L253 L291 L292 | L204 A3 L292 A13 | A3 L257 L292 | L253 L257 L291 L292 | L204 L254 L292 A13 | L40 L286 L287 L290 | L220 L221 L254 L256 L287 L288 L290 L291 | L40 L269 L270 L290 | L96 L268 L269 L290 | L170 L242 L244 L291 | L40 L283 L284 L290 | L211 L284 L285 L290 | A3 L253 L291 | A3 L257 L291 L292 | A3 L291 L292 A13 | A3 L253 L257 L291 | L254 L291 L292 A13 | L254 L256 L291 L292 | L193 L255 L256 L292 | L40 L285 L286 L290 | L217 L286 L287 L290 | L223 L255 L256 L291 | L40 L284 L285 L290 | L162 L187 L253 L257 L285 L286 L290 A13 | L162 L187 A3 L253 L257 A13 | A3 L257 L291 | L183 L254 L291 A13 | L255 L256 L291 L292 | L183 A3 L291 A13 | A5 | A6 | A7 | A8 | A9 makes body 1
extrude "Extrude10" add sketch "Base Sketch" against normal blind 3 contours L249 L295 L296 L298 | L262 L295 L296 L298 | L249 L261 L295 L296 | L248 L262 L295 L296 | L72 L248 L262 L296 L297 | L43 L248 L262 L297 | L261 L295 L296 L299 | L94 L135 L249 L261 L295 A12 | L125 L148 L248 L262 L294 L295 | L248 L263 L295 L296 | L43 L250 L260 L297 | L68 L250 L260 L296 L297 | L43 L248 L263 L297 | L250 L295 L296 L299 | L247 L263 L295 L296 | L85 L89 L247 L263 L296 L297 | L250 L260 L295 L296 | L43 L251 L260 L297 | L43 L247 L263 L297 | L75 L103 L247 L263 L294 L295 | L247 L264 L295 L296 | L54 L61 L250 L260 L294 L295 | L251 L260 L295 L296 | L43 L251 L259 L297 | L73 L87 L251 L259 L296 L297 | L43 L247 L264 L297 | L248 L262 L293 L294 | L262 L293 L294 A12 | L246 L264 L295 L296 | L45 L84 L246 L264 L296 L297 | L251 L259 L295 L296 | L43 L252 L259 L297 | L43 L246 L264 L297 | L153 L169 L248 L262 L292 L293 | L248 L263 L293 L294 | L50 L105 L246 L264 L294 L295 | L246 L265 L295 L296 | L108 L146 L251 L259 L294 L295 | L252 L259 L295 L296 | L43 L252 L258 L297 | L76 L90 L252 L258 L296 L297 | L43 L246 L265 L297 | L250 L293 L294 A12 | L247 L263 L293 L294 | L245 L265 L295 L296 | L38 L66 L245 L265 L296 L297 | L250 L260 L293 L294 | L252 L258 L295 L296 | L43 L253 L258 L297 | L43 L245 L265 L297 | L155 L209 L247 L263 L292 L293 | L247 L264 L293 L294 | L71 L92 L245 L265 L294 L295 | L245 L295 L296 A11 | L95 L171 L250 L260 L292 L293 | L251 L260 L293 L294 | L121 L147 L252 L258 L294 L295 | L253 L258 L295 L296 | L43 L253 L257 L297 | L59 L123 L253 L257 L296 L297 | L43 L245 L266 L297 | L98 L161 L249 L261 L292 A12 | L248 L262 L291 L292 | L249 L262 L291 L292 | L246 L264 L293 L294 | L251 L259 L293 L294 | L253 L257 L295 L296 | L43 L254 L257 L297 | L65 L86 L244 L266 L297 A11 | L43 L244 L266 L297 | L249 L261 L291 L292 | L130 L165 L248 L262 L275 L276 L290 L291 | L248 L263 L291 L292 | L132 L166 L246 L264 L292 L293 | L246 L265 L293 L294 | L180 L194 L251 L259 L292 L293 | L252 L259 L293 L294 | L104 L118 L253 L257 L294 L295 | L257 L295 L296 A14 | L43 L254 L256 L297 | L52 L60 L254 L256 L297 A14 | L43 L242 L244 L297 | L100 L189 L249 L261 L277 L278 L290 L291 | L250 L261 L291 L292 | L247 L263 L291 L292 | L245 L265 L293 L294 | L250 L260 L291 L292 | L252 L258 L293 L294 | L43 L255 L256 L297 | L10 L35 L40 L43 L106 L152 L173 L242 L243 | L99 L202 L247 L263 L273 L274 L290 L291 | L247 L264 L291 L292 | L117 L158 L245 L265 L293 A10 | L245 L266 L293 L294 | L143 L145 L244 L266 L294 A11 | L175 L199 L250 L260 L279 L280 L290 L291 | L251 L260 L291 L292 | L110 L168 L252 L258 L292 L293 | L253 L258 L293 L294 | L15 L40 L43 L114 L138 L203 L206 L255 L289 | L40 L275 L276 L290 | L40 L276 L277 L290 | L246 L264 L291 L292 | L244 L266 L293 L294 | L251 L259 L291 L292 | L253 L257 L293 L294 | L40 L277 L278 L290 | L40 L274 L275 L290 | L214 L218 L246 L264 L271 L272 L290 L291 | L246 L291 L292 A10 | L91 L134 L244 L266 L292 L293 | L242 L244 L293 L294 | L242 L295 L296 A11 | L182 L197 L251 L259 L281 L282 L290 L291 | L252 L259 L291 L292 | L172 L185 L253 L257 L293 A13 | L254 L257 L293 L294 | L128 L144 L254 L256 L294 A14 | L40 L278 L279 L290 | L40 L273 L274 L290 | L40 L279 L280 L290 | L252 L258 L291 L292 | L254 L256 L293 L294 | L255 L295 L296 A14 | L40 L243 L267 L290 | L40 L272 L273 L290 | L40 L280 L281 L290 | L176 L219 L252 L258 L283 L284 L290 L291 | L258 L291 L292 A13 | L163 L212 L254 L256 L292 L293 | L255 L256 L293 L294 | L40 L288 L289 L290 | L40 L267 L268 L290 | L40 L271 L272 L290 | L266 L291 L292 A10 | L244 L266 L291 L292 | L40 L281 L282 L290 | L40 L287 L288 L290 | L40 L268 L269 L290 | L159 L210 L244 L266 L267 L268 L290 L291 | L40 L270 L271 L290 | L174 L207 L245 L265 L269 L270 L290 A10 | L242 L244 L291 L292 | L40 L282 L283 L290 | L40 L286 L287 L290 | L220 L221 L254 L256 L287 L288 L290 L291 | L40 L269 L270 L290 | L40 L283 L284 L290 | L254 L291 L292 A13 | L254 L256 L291 L292 | L40 L285 L286 L290 | L40 L284 L285 L290 | L162 L187 L253 L257 L285 L286 L290 A13 | L255 L256 L291 L292 bodies 1
extrude "Extrude2" add sketch "Base Sketch" along normal blind 1 separate body contours L0 L1 L2 L3 L4 L5 L6 L7 L8 L9 L11 L13 L14 L16 L17 L18 L19 L20 L21 L22 L23 L24 L25 L26 L31 L36 L37 L41 L49 L56 L63 L67 L74 L79 L81 L82 | L0 L1 L2 L5 L6 L8 L14 L16 L17 L18 L21 L25 L36 L49 L67 L79 L82 L262 L296 L297 L298 L301 | L13 L249 L296 L298 | L3 L297 L300 L301 | L13 L249 L261 L296 | L249 L295 L296 L298 | L262 L295 L296 L298 | L4 L7 L9 L11 L19 L20 L22 L23 L24 L26 L31 L37 L41 L56 L63 L74 L81 L250 L296 L297 L299 L300 | L43 L262 L297 L301 | L43 L297 L300 L301 | L13 L261 L296 L299 | L249 L261 L295 L296 | L248 L262 L295 L296 | L72 L248 L262 L296 L297 | L120 L249 L295 L298 | L120 L262 L295 L298 | L43 L250 L297 L300 | L43 L248 L262 L297 | L261 L295 L296 L299 | L94 L135 L249 L261 L295 A12 | L125 L148 L248 L262 L294 L295 | L248 L263 L295 L296 | L51 L248 L263 L296 | L93 L120 L135 L148 L249 L262 A12 | L43 L250 L260 L297 | L68 L250 L260 L296 L297 | L69 L248 L263 L297 | L43 L248 L263 L297 | L250 L295 L296 L299 | L122 L261 L295 L299 | L124 L248 L263 L295 | L51 L69 L72 L85 L248 L263 | L247 L263 L295 L296 | L85 L89 L247 L263 L296 L297 | L250 L260 L295 L296 | L43 L251 L260 L297 | L28 L251 L260 L297 | L43 L247 L263 L297 | L122 L250 L295 L299 | L47 L61 L94 L122 L250 L261 A12 | L93 L135 L249 A12 | L94 L135 A1 L249 L261 A12 | L93 L262 L294 A12 | L103 L124 L125 L149 L248 L263 | L75 L103 L247 L263 L294 L295 | L247 L264 L295 L296 | L39 L247 L264 L296 | L54 L61 L250 L260 L294 L295 | L44 L251 L260 L296 | L251 L260 L295 L296 | L28 L44 L68 L87 L251 L260 | L43 L251 L259 L297 | L73 L87 L251 L259 L296 L297 | L80 L247 L264 L297 | L43 L247 L264 L297 | L47 L94 L261 A12 | A1 L249 L261 L294 | L93 A1 L294 A12 | A1 L249 L294 | L248 L262 L293 L294 | L262 L293 L294 A12 | L149 L248 L263 L294 | L53 L247 L264 L295 | L39 L45 L80 L89 L247 L264 | L246 L264 L295 L296 | L45 L84 L246 L264 L296 L297 | L48 L251 L260 L295 | L251 L259 L295 L296 | L43 L252 L259 L297 | L46 L252 L259 L297 | L43 L246 L264 L297 | L47 A1 L294 A12 | A1 L261 L294 | L47 L250 L294 A12 | A1 L293 L294 A12 | A1 L249 L293 L294 | L249 L261 L293 L294 | L153 L169 L248 L262 L292 L293 | L188 L262 L293 A12 | L248 L263 L293 L294 | L53 L75 L78 L105 L247 L264 | L50 L105 L246 L264 L294 L295 | L246 L265 L295 L296 | L88 L246 L265 L296 | L48 L54 L108 L154 L251 L260 | L108 L146 L251 L259 L294 L295 | L27 L252 L259 L296 | L252 L259 L295 L296 | L27 L46 L73 L76 L252 L259 | L43 L252 L258 L297 | L76 L90 L252 L258 L296 L297 | L77 L246 L265 L297 | L43 L246 L265 L297 | A1 L261 L293 L294 | A1 L293 L294 A12 | L250 L293 L294 A12 | L188 A1 L293 A12 | A1 L249 L293 | A1 L249 L261 L293 | L161 L169 L188 L213 L249 L262 A12 | L195 L248 L263 L293 | L247 L263 L293 L294 | L78 L247 L264 L294 | L64 L246 L265 L295 | L66 L77 L84 L88 L246 L265 | L245 L265 L295 L296 | L38 L66 L245 L265 L296 L297 | L250 L260 L293 L294 | L154 L251 L260 L294 | L113 L252 L259 L295 | L252 L258 L295 L296 | L43 L253 L258 L297 | L42 L253 L258 L297 | L43 L245 L265 L297 | A1 L261 L293 | L161 L188 L249 A12 | L98 L161 A1 L249 L261 A12 | L213 L249 L262 L292 | L153 L179 L195 L209 L248 L263 | L155 L209 L247 L263 L292 L293 | L247 L264 L293 L294 | L33 L50 L64 L92 L246 L265 | L71 L92 L245 L265 L294 L295 | L245 L295 L296 A11 | L83 L245 L296 A11 | L190 L250 L293 A12 | L95 L171 L250 L260 L292 L293 | L251 L260 L293 L294 | L97 L113 L121 L146 L252 L259 | L121 L147 L252 L258 L294 L295 | L70 L253 L258 L296 | L253 L258 L295 L296 | L42 L59 L70 L90 L253 L258 | L43 L253 L257 L297 | L59 L123 L253 L257 L296 L297 | L29 L245 L266 L297 | L43 L245 L266 L297 | L190 A1 L293 A12 | L98 L190 L261 A12 | L98 L161 L249 L261 L292 A12 | L248 L262 L291 L292 | L249 L262 L291 L292 | L179 L248 L263 L292 | L129 L247 L264 L293 | L246 L264 L293 L294 | L33 L246 L265 L294 | L107 L245 L295 A11 | L29 L38 L83 L86 L245 L266 A11 | L83 A2 L296 A11 | A2 L295 L296 A11 | L95 L98 L190 L191 L250 L261 A12 | L142 L251 L260 L293 | L251 L259 L293 L294 | L97 L252 L259 L294 | L115 L253 L258 L295 | L253 L257 L295 L296 | L43 L254 L257 L297 | L141 L254 L257 L297 | L65 L86 L244 L266 L297 A11 | L43 L244 L266 L297 | L249 L261 L291 L292 | L130 L165 L248 L262 L275 L276 L290 L291 | L167 L249 L262 L291 | L248 L263 L291 L292 | L127 L129 L155 L166 L247 L264 | L132 L166 L246 L264 L292 L293 | L246 L265 L293 L294 | L32 L71 L107 L145 L245 L266 A11 | L107 A2 L295 A11 | L83 L86 L266 A11 | A2 L266 L295 L296 | A2 L266 L296 | L191 L250 L261 L292 | L142 L156 L171 L194 L251 L260 | L180 L194 L251 L259 L292 L293 | L252 L259 L293 L294 | L102 L115 L118 L147 L253 L258 | L104 L118 L253 L257 L294 L295 | L58 L257 L296 A14 | L257 L295 L296 A14 | L52 L58 L123 L141 L254 L257 A14 | L43 L254 L256 L297 | L52 L60 L254 L256 L297 A14 | L57 L242 L244 L297 | L43 L242 L244 L297 | L100 L189 L249 L261 L277 L278 L290 L291 | L250 L261 L291 L292 | L100 L151 L165 L167 L249 L262 | L112 L248 L263 L291 | L247 L263 L291 L292 | L127 L247 L264 L292 | L205 L246 L265 L293 | L245 L265 L293 L294 | L32 L245 L266 L294 | L107 L145 L266 A11 | A2 L266 L295 | L65 L86 A2 L244 L266 A11 | A2 L244 L266 L296 | L244 L266 L295 L296 | L250 L260 L291 L292 | L156 L251 L260 L292 | L216 L252 L259 L293 | L252 L258 L293 L294 | L102 L253 L258 L294 | L55 L257 L295 A14 | A0 L295 L296 A14 | L58 A0 L296 A14 | L43 L255 L256 L297 | L30 L255 L256 L297 | L12 L35 L57 L65 L242 L244 A11 | L10 L35 L40 L43 L106 L152 L173 L242 L243 | L196 L250 L261 L291 | L151 L276 L277 L290 | L99 L111 L112 L130 L248 L263 | L99 L202 L247 L263 L273 L274 L290 L291 | L247 L264 L291 L292 | L132 L150 L158 L205 L246 L265 A10 | L117 L158 L245 L265 L293 A10 | L245 L266 L293 L294 | L143 L145 L244 L266 L294 A11 | L143 L145 A2 L244 L266 A11 | A2 L244 L266 L295 | L12 L65 L244 A11 | L12 A2 L296 A11 | A2 L244 L296 | A2 L244 L295 L296 | L175 L199 L250 L260 L279 L280 L290 L291 | L251 L260 L291 L292 | L101 L110 L180 L216 L252 L259 | L110 L168 L252 L258 L292 L293 | L253 L258 L293 L294 | L55 L104 L128 L137 L254 L257 A14 | L55 A0 L295 A14 | L52 L58 L254 A14 | A0 L254 L296 | A0 L254 L295 L296 | L52 L60 A0 L254 L256 A14 | L30 L60 L62 L138 L255 L256 A14 | L15 L40 L43 L114 L138 L203 L206 L255 L289 | L175 L189 L196 L201 L250 L261 | L40 L275 L276 L290 | L40 L276 L277 L290 | L111 L274 L275 L290 | L126 L247 L264 L291 | L246 L264 L291 L292 | L150 L246 L292 A10 | L116 L245 L266 L293 | L244 L266 L293 L294 | L34 A2 L295 A11 | L34 L143 L244 A11 | A2 L244 L295 | L34 L106 L140 L143 L242 L244 A11 | L12 L242 L296 A11 | A2 L295 L296 A11 | L178 L251 L260 L291 | L251 L259 L291 L292 | L101 L252 L259 L292 | L198 L253 L258 L293 | L253 L257 L293 L294 | L55 L128 L254 A14 | L137 L254 L257 L294 | A0 L254 L295 | A0 L254 L256 L296 | L254 L256 L295 L296 | L60 L62 L256 A14 | L40 L277 L278 L290 | L201 L278 L279 L290 | L40 L274 L275 L290 | L126 L157 L202 L214 L247 L264 | L214 L218 L246 L264 L271 L272 L290 L291 | L246 L291 L292 A10 | L150 L158 L265 A10 | L150 A4 L292 A10 | L117 L158 A4 L245 L265 A10 | L91 L116 L117 L119 L245 L266 A10 | L91 L134 L244 L266 L292 L293 | L242 L244 L293 L294 | L140 L242 L244 L294 | L34 L242 L295 A11 | L242 L295 L296 A11 | L178 L182 L199 L200 L251 L260 | L182 L197 L251 L259 L281 L282 L290 L291 | L252 L259 L291 L292 | L168 L185 L192 L198 L253 L258 A13 | L172 L185 L253 L257 L293 A13 | L254 L257 L293 L294 | L128 L144 A0 L254 L256 A14 | A0 L254 L256 L295 | L128 L144 L254 L256 L294 A14 | L62 A0 L296 A14 | A0 L256 L296 | A0 L256 L295 L296 | L62 L255 L296 A14 | L40 L278 L279 L290 | L40 L273 L274 L290 | L157 L272 L273 L290 | L181 L246 L291 A10 | A4 L291 L292 A10 | A4 L265 L292 | A4 L245 L265 L292 | L117 L119 L245 A10 | L136 L242 L244 L293 | L40 L279 L280 L290 | L200 L280 L281 L290 | L215 L252 L259 L291 | L252 L258 L291 L292 | L192 L258 L292 A13 | L184 L254 L257 L293 | L254 L256 L293 L294 | L133 L144 L256 A14 | L133 A0 L295 A14 | A0 L256 L295 | L114 L133 L139 L144 L255 L256 A14 | A0 L295 L296 A14 | L255 L295 L296 A14 | L40 L243 L267 L290 | L40 L272 L273 L290 | L131 L174 L181 L218 L246 L265 A10 | L181 A4 L291 A10 | A4 L265 L291 L292 | L119 A4 L292 A10 | A4 L245 L292 | L245 L265 L291 L292 | L119 L266 L292 A10 | L109 L134 L136 L152 L242 L244 | L40 L280 L281 L290 | L197 L215 L219 L222 L252 L259 | L176 L219 L252 L258 L283 L284 L290 L291 | L258 L291 L292 A13 | L192 A3 L292 A13 | L185 L192 L253 A13 | L172 L185 A3 L253 L257 A13 | L172 L184 L204 L212 L254 L257 A13 | L163 L212 L254 L256 L292 L293 | L139 L255 L256 L294 | L255 L256 L293 L294 | L133 L255 L295 A14 | L40 L288 L289 L290 | L40 L267 L268 L290 | L164 L243 L267 L290 | L40 L271 L272 L290 | L174 L181 L265 A10 | L131 L270 L271 L290 | A4 L265 L291 | A4 L291 L292 A10 | A4 L245 L291 L292 | A4 L245 L265 L291 | L266 L291 L292 A10 | L244 L266 L291 L292 | L109 L242 L244 L292 | L40 L281 L282 L290 | L222 L282 L283 L290 | L208 L258 L291 A13 | A3 L291 L292 A13 | A3 L253 L257 L292 | A3 L253 L292 | L172 L204 L257 A13 | L186 L255 L256 L293 | L40 L287 L288 L290 | L160 L288 L289 L290 | L40 L268 L269 L290 | L159 L210 L244 L266 L267 L268 L290 L291 | L164 L170 L173 L210 L242 L244 | L40 L270 L271 L290 | L174 L207 A4 L245 L265 A10 | L174 L207 L245 L265 L269 L270 L290 A10 | L177 A4 L291 A10 | A4 L245 L291 | L177 L266 L291 A10 | L242 L244 L291 L292 | L40 L282 L283 L290 | L176 L187 L208 L211 L253 L258 A13 | L208 A3 L291 A13 | A3 L253 L291 L292 | L204 A3 L292 A13 | A3 L257 L292 | L253 L257 L291 L292 | L204 L254 L292 A13 | L163 L186 L193 L203 L255 L256 | L40 L286 L287 L290 | L220 L221 L254 L256 L287 L288 L290 L291 | L160 L206 L220 L223 L255 L256 | L40 L269 L270 L290 | L96 L268 L269 L290 | L170 L242 L244 L291 | L177 L207 L245 A10 | L96 L159 L177 L207 L245 L266 A10 | L40 L283 L284 L290 | L211 L284 L285 L290 | L187 L208 L253 A13 | A3 L253 L291 | A3 L257 L291 L292 | A3 L291 L292 A13 | A3 L253 L257 L291 | L254 L291 L292 A13 | L254 L256 L291 L292 | L193 L255 L256 L292 | L40 L285 L286 L290 | L217 L286 L287 L290 | L223 L255 L256 L291 | L40 L284 L285 L290 | L162 L187 L253 L257 L285 L286 L290 A13 | L162 L187 A3 L253 L257 A13 | A3 L257 L291 | L183 L254 L291 A13 | L255 L256 L291 L292 | L162 L183 L217 L221 L254 L257 A13 | L162 L183 L257 A13 | L183 A3 L291 A13 | L224 L225 L226 L227 | L228 L229 L230 L231 | A5 | A6 | A7 | A8 | A9 makes body 2
extrude "Extrude3" add sketch "Base Sketch" along normal blind 18 contours L228 L229 L230 L231 bodies 2
extrude "Extrude4" add sketch "Base Sketch" along normal blind 11 contours A1 L249 L261 L294 | A1 L249 L294 | A1 L261 L294 | A1 L249 L293 L294 | L249 L261 L293 L294 | A1 L261 L293 L294 | A1 L249 L293 | A1 L249 L261 L293 | A1 L261 L293 | A2 L266 L295 L296 | A2 L266 L296 | A2 L266 L295 | A2 L244 L266 L296 | L244 L266 L295 L296 | A2 L244 L266 L295 | A2 L244 L296 | A2 L244 L295 L296 | A0 L254 L296 | A0 L254 L295 L296 | A2 L244 L295 | A0 L254 L295 | A0 L254 L256 L296 | L254 L256 L295 L296 | A0 L254 L256 L295 | A0 L256 L296 | A0 L256 L295 L296 | A4 L265 L292 | A4 L245 L265 L292 | A0 L256 L295 | A4 L265 L291 L292 | A4 L245 L292 | L245 L265 L291 L292 | A4 L265 L291 | A4 L245 L291 L292 | A4 L245 L265 L291 | A3 L253 L257 L292 | A3 L253 L292 | A4 L245 L291 | A3 L253 L291 L292 | A3 L257 L292 | L253 L257 L291 L292 | A3 L253 L291 | A3 L257 L291 L292 | A3 L253 L257 L291 | A3 L257 L291 | A5 | A6 | A7 | A8 | A9 bodies 2
sketch "Sketch2" plane through (0, 0, 1) normal (0, 0, 1) x (-1, 0, 0)
  circle A0 centre (-190.5945, -57.4085) radius 3.5715
  circle A1 centre (-114.3935, -38.3584) radius 3.5708
  circle A2 centre (-38.1944, -57.4085) radius 3.5714
  circle A3 centre (-19.1445, -19.3084) radius 3.5712
  circle A4 centre (-209.6445, -19.3084) radius 3.5714
  line L0 (-228.995, 0.0423) -> (-228.995, -76.7575)
  line L1 (-228.995, -76.7575) -> (0.2049, -76.7575)
  line L2 (0.2049, -76.7575) -> (0.2049, 0.0423)
  line L3 (0.2049, 0.0423) -> (-228.995, 0.0423)
  line L4 (-3.47, -76.7575) -> (-23.47, -76.7575)
  line L5 (-23.47, -76.7575) -> (-23.47, -41.7575)
  line L6 (-23.47, -41.7575) -> (-3.47, -41.7575)
  line L7 (-3.47, -41.7575) -> (-3.47, -76.7575)
  line L8 (-1.6912, -76.7575) -> (-25.1457, -76.7575)
  line L9 (-25.1457, -76.7575) -> (-25.1457, -40)
  line L10 (-25.1457, -40) -> (-1.6912, -40)
  line L11 (-1.6912, -40) -> (-1.6912, -76.7575)
  dimension "d19" = 20
  dimension "d20" = 35
  constraint horizontal L4
  constraint vertical L5
  constraint horizontal L6
  constraint vertical L7
  constraint coincident L1 L4.start
  constraint horizontal L8
  constraint vertical L9
  constraint horizontal L10
  constraint vertical L11
  constraint coincident L1 L8.start
  measures "d19" distance of L4.start L4.end
  measures "d20" distance of L4.start L6.end
extrude "Extrude5" add sketch "Sketch2" along normal blind 1.5 contours L1 L5 L6 L7 L8 L9 L10 L11 bodies 2
sketch "Sketch3" plane through (0, 76.7575, 0) normal (0, -1, 0) x (1, 0, 0)
  line L0 (23.47, 1) -> (23.47, 2.5)
  line L1 (23.47, 2.5) -> (25.1457, 2.5)
  line L2 (25.1457, 2.5) -> (25.1457, 1)
  line L3 (25.1457, 1) -> (228.995, 1)
  line L4 (228.995, 1) -> (228.995, 18)
  line L5 (228.995, 18) -> (-0.2049, 18)
  line L6 (-0.2049, 18) -> (-0.2049, 1)
  line L7 (-0.2049, 1) -> (1.6912, 1)
  line L8 (1.6912, 1) -> (1.6912, 2.5)
  line L9 (1.6912, 2.5) -> (3.47, 2.5)
  line L10 (3.47, 2.5) -> (3.47, 1)
  line L11 (3.47, 1) -> (23.47, 1)
  line L12 (8.97, 6.2) -> (17.97, 6.2)
  line L13 (17.97, 6.2) -> (17.97, 3)
  line L14 (17.97, 3) -> (8.97, 3)
  line L15 (8.97, 3) -> (8.97, 6.2)
  circle A0 centre (10.57, 4.6) radius 1.6
  circle A1 centre (16.37, 4.6) radius 1.6
  line L16 (3.47, 1) -> (3.47, 18) construction
  line L17 (23.47, 1) -> (23.47, 18) construction
  line L18 (3.47, 3) -> (23.47, 3) construction
  dimension "d23" = 9
  dimension "d24" = 3.2
  dimension "d60" = 2
  constraint horizontal L12
  constraint vertical L13
  constraint horizontal L14
  constraint vertical L15
  constraint tangent L14 A0
  constraint tangent L14 A1
  constraint tangent L12 A1
  constraint tangent L13 A1
  constraint tangent L15 A0
  constraint tangent L12 A0
  constraint coincident L10.end L11.start
  constraint coincident L5 L16.end
  constraint perpendicular L5 L16
  constraint coincident L0.start L11.end
  constraint coincident L5 L17.end
  constraint perpendicular L5 L17
  constraint coincident L16 L18.start
  constraint coincident L17 L18.end
  constraint perpendicular L17 L18
  constraint midpoint L14 L18
  measures "d23" distance of L12.start L12.end
  measures "d24" distance of L12.start L14.end
  measures "d60" distance of L11 L18
extrude "Extrude6" cut sketch "Sketch3" against normal blind 12.5 contours L12 L14 A0 A1 | A0 | A1 bodies 2
fillet "Fillet1" radius 2.5 4 edges at (-2.0049, 78.5575, 9) (-2.0049, -1.8423, 9) (230.795, 78.5575, 9) (230.795, -1.8423, 9) on bodies 2
fillet "Fillet3" radius 1.5 8 edges at (230.0628, 77.8253, 0) (230.795, 38.3576, 0) (230.0628, -1.1101, 0) (114.395, -1.8423, 0) (-1.2727, -1.1101, 0) (-2.0049, 38.3576, 0) (-1.2727, 77.8253, 0) (114.395, 78.5575, 0) on bodies 2
fillet "Fillet4" radius 0.75 4 edges at (228.995, -0.0423, 9.5) (228.995, 76.7575, 9.5) (-0.2049, -0.0423, 9.5) (-0.2049, 76.7575, 9.5) on bodies 2
fillet "Fillet5" radius 0.9 16 edges at (-1.2727, 77.8253, 18) (114.395, 78.5575, 18) (230.0628, 77.8253, 18) (230.795, 38.3576, 18) (230.0628, -1.1101, 18) (114.395, -1.8423, 18) (-1.2727, -1.1101, 18) (-2.0049, 38.3576, 18) (228.7753, 76.5378, 18) (114.395, 76.7575, 18) (0.0148, 76.5378, 18) (-0.2049, 38.3576, 18) (0.0148, 0.1774, 18) (114.395, -0.0423, 18) (228.7753, 0.1774, 18) (228.995, 38.3576, 18) on bodies 2
move_body "Move2" bodies 2 to x (1, 0, 0) y (0, 1, 0) z (0, 0, 1) at (0, 0, -11)
extrude "Extrude8" cut sketch "Base Sketch" along normal blind 10 and the other way blind 9 contours A5 | A6 | A7 | A8 | A9 bodies 1 2
chamfer "Chamfer1" distance 1 angle 45 5 edges at (37.262, 57.7701, 1.6) (18.2121, 19.67, 1.6) (113.4612, 38.72, 1.6) (208.7122, 19.67, 1.6) (189.6622, 57.7701, 1.6) on bodies 1